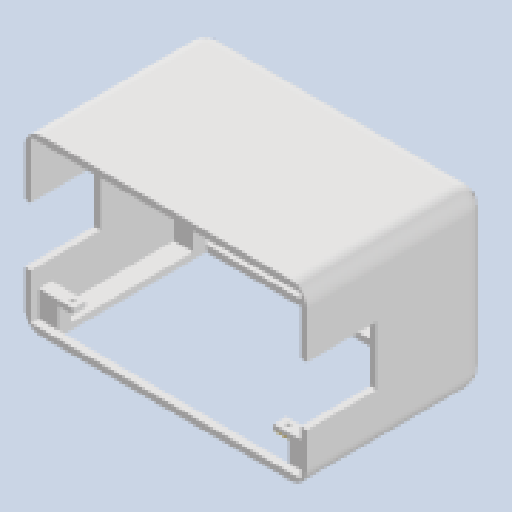
# Autodesk Inventor part: лицо
Saved by Autodesk Inventor 2024.2 (Build 282272000, 272)
## iProperties
Created: 2025-10-19
Part Number: лицо
Material: Типовые
Document SubType Name: Modeling
Designer: katya_notebook
Density: 1 g/cm^3
Appearance: По умолчанию
Author: katya_notebook
Autodesk Inventor part; units mm, degrees
ref_plane "YZ Plane" through (0, 0, 0) normal (1, 0, 0) x (0, 1, 0)
ref_plane "XZ Plane" through (0, 0, 0) normal (0, 1, 0) x (-1, 0, 0)
ref_plane "XY Plane" through (0, 0, 0) normal (0, 0, 1) x (1, 0, 0)
sketch "Эскиз1" plane through (0, 0, 0) normal (0, 0, 1) x (1, 0, 0)
  line L0 (-65, -40) -> (65, -40)
  line L1 (65, -40) -> (65, 40)
  line L2 (65, 40) -> (-65, 40)
  line L3 (-65, 40) -> (-65, -40)
  line L4 (-65, -40) -> (65, 40) construction
  line L5 (65, -40) -> (-65, 40) construction
  point P0 (0, 0)
  dimension "d0" = 80
  dimension "d1" = 130
  constraints: 12 end point, 2 midpoint, 2 parallel, 1 horizontal, 1 perpendicular
  measures "d0" distance of L0.end L1.end
  measures "d1" distance of L1.end L2.end
extrude "Выдавливание1" add sketch "Эскиз1" along normal blind 3
sketch "Эскиз2" plane through (0, 0, 3) normal (0, 0, 1) x (1, 0, 0)
  line L0 (-62, -37) -> (62, -37)
  line L1 (62, -37) -> (62, 37)
  line L2 (62, 37) -> (-62, 37)
  line L3 (-62, 37) -> (-62, -37)
  line L4 (-62, -37) -> (62, 37) construction
  line L5 (62, -37) -> (-62, 37) construction
  line L6 (-65, -40) -> (65, -40)
  line L7 (65, -40) -> (65, 40)
  line L8 (65, 40) -> (-65, 40)
  line L9 (-65, 40) -> (-65, -40)
  line L10 (-65, -40) -> (65, 40) construction
  line L11 (65, -40) -> (-65, 40) construction
  point P0 (0, 0)
  dimension "d8" = 3
  dimension "d9" = 3
  constraints: 24 end point, 4 midpoint, 4 parallel, 2 horizontal, 2 perpendicular
  measures "d8" distance between parallel lines of L7 L1
  measures "d9" distance between parallel lines of L2 L8
extrude "Выдавливание2" add sketch "Эскиз2" along normal blind 80
fillet "Сопряжение1" radius 8 8 edges at (-65, 40, 41.5) (-65, -40, 41.5) (65, -40, 41.5) (65, 40, 41.5) (-65, 0, 0) (0, -40, 0) (65, 0, 0) (0, 40, 0)
sketch "Эскиз3" plane through (-57, -40, 8) normal (0, -1, 0) x (1, 0, 0)
  line L0 (110, 71.5) -> (4, 71.5) projected
  line L1 (4, 71.5) -> (4, 3.5) projected
  line L2 (4, 71.5) -> (110, 71.5)
  line L3 (4, 3.36) -> (4, 71.5)
  line L4 (57, 71.5) -> (57, 3.5)
  line L5 (4, 37.43) -> (110.34, 37.43)
  line L6 (110.34, 3.36) -> (4, 3.36)
  line L7 (4, 3.36) -> (4, 71.5)
  line L8 (4, 71.5) -> (110.34, 71.5)
  line L9 (110.34, 71.5) -> (110.34, 3.36)
  line L10 (110.34, 3.36) -> (4, 71.5) construction
  line L11 (4, 3.36) -> (110.34, 71.5) construction
  point P0 (57, -8)
  point P1 (57.17, 37.43)
  point P2 (4, 3.5)
  point P3 (4, 3.36)
  dimension "d16" = 106.34
  dimension "d17" = 68.14
  constraints: 20 end point, 5 midpoint, 2 horizontal, 2 parallel, 1 perpendicular
  measures "d16" distance of L6.start L6.end
  measures "d17" distance of L8.end L6.start
extrude "Выдавливание3" cut sketch "Эскиз3" against normal blind 12
sketch "Эскиз4" plane through (0, 0, 0) normal (0, 0, -1) x (-1, 0, 0)
  circle A0 centre (11.8725, 0) radius 2 projected
  circle A1 centre (-11.8725, 0) radius 2 projected
  line L0 (15, -19.9954) -> (-15, -19.9954) construction
  line L1 (15, -7.4954) -> (15, -19.9954) construction
  line L2 (-15, -7.4954) -> (15, -7.4954) construction
  line L3 (-15, -19.9954) -> (-15, -7.4954) construction
  circle A2 centre (11.8725, 0) radius 2
  circle A3 centre (-11.8725, 0) radius 2
  line L4 (-15, -7.4954) -> (15, -7.4954)
  line L5 (15, -7.4954) -> (15, -19.9954)
  line L6 (15, -19.9954) -> (-15, -19.9954)
  line L7 (-15, -19.9954) -> (-15, -7.4954)
  line L8 (-15, -7.4954) -> (15, -19.9954) construction
  line L9 (15, -7.4954) -> (-15, -19.9954) construction
  line L10 (20.0944, 0) -> (-19.4677, 0)
  line L11 (15, 19.9954) -> (-15, 19.9954) construction
  line L12 (15, 7.4954) -> (15, 19.9954) construction
  line L13 (-15, 7.4954) -> (15, 7.4954) construction
  line L14 (-15, 19.9954) -> (-15, 7.4954) construction
  line L15 (-15, 19.9954) -> (15, 19.9954)
  line L16 (15, 19.9954) -> (15, 7.4954)
  line L17 (15, 7.4954) -> (-15, 7.4954)
  line L18 (-15, 7.4954) -> (-15, 19.9954)
  line L19 (-15, 19.9954) -> (15, 7.4954) construction
  line L20 (15, 19.9954) -> (-15, 7.4954) construction
  point P0 (0, 0)
  point P1 (0, -13.7454)
  point P2 (0, 13.7454)
  constraints: 34 end point, 4 midpoint, 4 parallel, 4 symmetric about line, 3 horizontal, 2 centre point, 2 coincident, 2 concentric, 2 perpendicular
extrude "Выдавливание4" cut sketch "Эскиз4" against normal blind 10
sketch "Эскиз5" plane through (-62, -37, 3) normal (0, 1, 0) x (1, 0, 0)
  circle A0 centre (111.7, -73.45) radius 2.75 projected
  circle A1 centre (12.5, -73.45) radius 2.75 projected
  circle A2 centre (111.7, -11.55) radius 2.75 projected
  circle A3 centre (12.5, -11.55) radius 2.75 projected
  line L0 (115.2, -76.5) -> (115.2, -8.5) projected
  line L1 (9, -8.5) -> (9, -76.5) projected
  line L2 (115.34, -76.5) -> (9, -76.5) projected
  line L3 (115.34, -8.36) -> (115.34, -76.5) projected
  line L4 (115.34, -76.5) -> (125.34, -76.5)
  line L5 (125.34, -76.5) -> (125.34, -70.5)
  line L6 (125.34, -70.5) -> (115.34, -70.5)
  line L7 (115.34, -70.5) -> (115.34, -76.5)
  line L8 (9, -8.36) -> (115.34, -8.36) projected
  line L9 (115.34, -8.36) -> (125.34, -8.36)
  line L10 (125.34, -8.36) -> (125.34, -14.36)
  line L11 (125.34, -14.36) -> (115.34, -14.36)
  line L12 (115.34, -14.36) -> (115.34, -8.36)
  line L13 (9, -76.5) -> (-1, -76.5)
  line L14 (-1, -76.5) -> (-1, -70.5)
  line L15 (-1, -70.5) -> (9, -70.5)
  line L16 (9, -70.5) -> (9, -76.5)
  line L17 (9, -76.5) -> (9, -8.36) projected
  line L18 (9, -8.36) -> (-1, -8.36)
  line L19 (-1, -8.36) -> (-1, -14.36)
  line L20 (-1, -14.36) -> (9, -14.36)
  line L21 (9, -14.36) -> (9, -8.36)
  point P0 (62, 3)
  point P1 (9, -14.36)
  point P2 (9, -70.5)
  dimension "d20" = 6
  dimension "d21" = 10
  dimension "d22" = 10
  dimension "d23" = 6
  dimension "d24" = 6
  dimension "d25" = 10
  dimension "d26" = 10
  dimension "d27" = 6
  constraints: 32 end point, 8 parallel, 4 horizontal, 4 perpendicular
  measures "d20" distance of L4.end L5.end
  measures "d21" distance of L5.end L6.end
  measures "d22" distance of L10.end L11.end
  measures "d23" distance of L9.end L10.end
  measures "d24" distance of L13.end L14.end
  measures "d25" distance of L1.end L13.end
  measures "d26" distance of L19.end L20.end
  measures "d27" distance of L18.end L19.end
ref_plane "РабПлоскость1" through (-52.25, -27.4, 73.7) normal (0, 1, 0) x (0, 0, 1)
extrude "Выдавливание5" add sketch "Эскиз5" along normal up to surface (9.6 mm away) contours L1 L20 L19 L18 L17 | L1 L13 L14 L15 | L9 L10 L11 L3 | L6 L5 L4 L3
ref_plane "РабПлоскость2" through (0.1, -27.4, 2.5765) normal (0, 1, 0) x (1, 0, 0)
sketch "Эскиз6" plane through (0.1, -27.4, 2.5765) normal (0, 1, 0) x (1, 0, 0)
  circle A0 centre (49.6, -73.8735) radius 1 projected
  circle A1 centre (-49.6, -73.8735) radius 1 projected
  circle A2 centre (-49.6, -11.9735) radius 1 projected
  circle A3 centre (49.6, -11.9735) radius 1 projected
  line L0 (61.9, -76.9235) -> (53.24, -76.9235) projected
  line L1 (61.9, -70.9235) -> (61.9, -76.9235) projected
  line L2 (61.9, -76.9235) -> (45.9, -76.9235)
  line L3 (45.9, -76.9235) -> (45.9, -70.9235)
  line L4 (45.9, -70.9235) -> (61.9, -70.9235)
  line L5 (61.9, -70.9235) -> (61.9, -76.9235)
  circle A4 centre (49.6, -73.8735) radius 1
  line L6 (61.9, -14.7835) -> (53.24, -14.7835) projected
  line L7 (61.9, -8.7835) -> (61.9, -14.7835) projected
  line L8 (-53.1, -76.9235) -> (-62.1, -76.9235) projected
  line L9 (-62.1, -76.9235) -> (-62.1, -70.9235) projected
  line L10 (-62.1, -14.7835) -> (-62.1, -8.7835) projected
  line L11 (-53.1, -14.7835) -> (-62.1, -14.7835) projected
  line L12 (61.9, -14.7835) -> (45.9, -14.7835)
  line L13 (45.9, -14.7835) -> (45.9, -8.7835)
  line L14 (45.9, -8.7835) -> (61.9, -8.7835)
  line L15 (61.9, -8.7835) -> (61.9, -14.7835)
  circle A5 centre (49.6, -11.9735) radius 1
  circle A6 centre (-49.6, -73.8735) radius 1
  circle A7 centre (-49.6, -11.9735) radius 1
  line L16 (-62.1, -76.9235) -> (-46.1, -76.9235)
  line L17 (-46.1, -76.9235) -> (-46.1, -70.9235)
  line L18 (-46.1, -70.9235) -> (-62.1, -70.9235)
  line L19 (-62.1, -70.9235) -> (-62.1, -76.9235)
  line L20 (-62.1, -14.7835) -> (-46.1, -14.7835)
  line L21 (-46.1, -14.7835) -> (-46.1, -8.7835)
  line L22 (-46.1, -8.7835) -> (-62.1, -8.7835)
  line L23 (-62.1, -8.7835) -> (-62.1, -14.7835)
  point P0 (-0.1, 2.5765)
  point P1 (61.9, -8.7835)
  point P2 (61.9, -70.9235)
  point P3 (53.24, -76.9235)
  point P4 (-62.1, -70.9235)
  dimension "d30" = 16
  dimension "d31" = 16
  dimension "d32" = 6
  dimension "d33" = 16
  dimension "d34" = 16
  constraints: 32 end point, 8 parallel, 4 centre point, 4 coincident, 4 concentric, 4 horizontal, 4 perpendicular
  measures "d30" distance of L3.end L4.end
  measures "d31" distance of L13.end L14.end
  measures "d32" distance of L16.end L17.end
  measures "d33" distance of L17.end L18.end
  measures "d34" distance of L10.start L20.end
extrude "Выдавливание6" add sketch "Эскиз6" along normal blind 2.5
sketch "Эскиз7" plane through (65, -32, 83) normal (1, 0, 0) x (0, 0, -1)
  line L0 (6.631, 19.5) -> (-99.237, 19.5) projected
  line L1 (6.631, 39.5) -> (-99.237, 39.5) projected
  line L2 (-8, 16) -> (0, 16) projected
  line L3 (0, 43) -> (-8, 43) projected
  line L4 (-8, 16) -> (32, 16)
  line L5 (32, 16) -> (32, 43)
  line L6 (32, 43) -> (-8, 43)
  line L7 (-8, 16) -> (-8, 43)
  point P0 (83, 32)
  point P1 (0, 16)
  dimension "d39" = 40
  constraints: 8 end point, 2 perpendicular, 1 collinear, 1 horizontal
  measures "d39" distance of L2.start L4.end
extrude "Выдавливание7" cut sketch "Эскиз7" against normal blind 162
